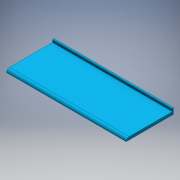
# Autodesk Inventor part: meson
Saved by Autodesk Inventor 2016 (Build 200138000, 138)
## iProperties
Created: 2015-11-25
Part Number: meson
Material: Generic
Document SubType Name: Modeling
Designer: Daniela
Density: 1 g/cm^3
Appearance: Exposed Aggregate - Warm Gray
Author: Daniela
Autodesk Inventor part; units mm, degrees
ref_plane "YZ Plane" through (0, 0, 0) normal (1, 0, 0) x (0, 1, 0)
ref_plane "XZ Plane" through (0, 0, 0) normal (0, 1, 0) x (-1, 0, 0)
ref_plane "XY Plane" through (0, 0, 0) normal (0, 0, 1) x (1, 0, 0)
sketch "Sketch1" plane through (0, 0, 0) normal (0, 0, 1) x (1, 0, 0)
  line L0 (0, 0) -> (1033.3333, 0)
  line L1 (1033.3333, 0) -> (1033.3333, 790)
  line L2 (1033.3333, 790) -> (0, 790)
  line L3 (0, 790) -> (0, 0)
  dimension "ancho" = 1033.3333
  dimension "d1" = 790
  constraints: 8 end point, 2 parallel, 1 horizontal, 1 perpendicular
  measures "ancho" distance of L1.end L2.end
  measures "d1" distance of L2.end L0.start
extrude "Extrusion1" add sketch "Sketch1" along normal blind 50
fillet "Fillet1" radius 50 1 edges at (516.6667, 0, 50)
sketch "Sketch2" plane through (1033.3333, 790, 50) normal (1, 0, 0) x (0, 0, -1)
  line L0 (50, 0) -> (-50, 0)
  line L1 (-50, 0) -> (-50, 0)
  line L2 (-30, -20) -> (50, -20)
  line L3 (50, -20) -> (50, 0)
  arc A0 (-50, 0) -> (-30, -20) centre (-30, 0) ccw
  point P0 (50, -790)
  point P1 (-50, -20)
  dimension "d5" = 100
  dimension "d6" = 20
  dimension "d7" = 20
  constraints: 8 end point, 2 parallel, 2 point on circle, 2 point on line, 2 tangent, 1 centre point, 1 horizontal, 1 perpendicular
  measures "d5" distance of point (-50, -20) L2.end
  measures "d6" distance of L0.end point (-50, -20)
  measures "d7" radius of A0
extrude "Extrusion2" add sketch "Sketch2" against normal up to surface (1033.3333 mm away)
body "Solid1"
